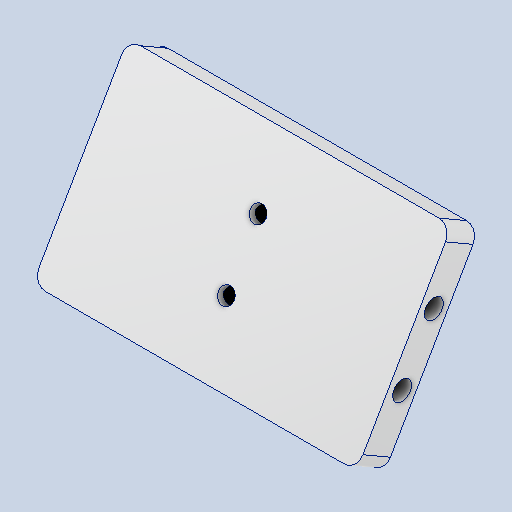
# Autodesk Inventor part: belt_liner_v5_Plate_4
Saved by Autodesk Inventor 2025.2 (Build 292293000, 293)
## iProperties
Created: 2025-02-23
Part Number: belt_liner_v5_Plate_4
Material: アルミニウム 6061
Document SubType Name: Modeling
Designer: haruy
Density: 2.7 g/cm^3
Appearance: アルミニウム - フラット
Author: haruy
Autodesk Inventor part; units mm, degrees
ref_plane "YZ Plane" through (0, 0, 0) normal (1, 0, 0) x (0, 1, 0)
ref_plane "XZ Plane" through (0, 0, 0) normal (0, 1, 0) x (-1, 0, 0)
ref_plane "XY Plane" through (0, 0, 0) normal (0, 0, 1) x (1, 0, 0)
derived "belt_liner_v5_Sketch_Base.ipt"
sketch "スケッチ1" plane through (300, 0, 0) normal (1, 0, 0) x (0, 1, 0)
  circle A0 centre (0, 0) radius 22.36
  circle A1 centre (742.4003, -428.625) radius 23.875 construction
  line L0 (0, 0) -> (0, -985.832)
  line L1 (0, 0) -> (742.4003, -428.625)
  line L2 (-48.7433, -24.4258) -> (-56.2433, -37.4162)
  line L3 (-56.2433, -37.4162) -> (725.7777, -488.9162)
  line L4 (725.7777, -488.9162) -> (733.2777, -475.9258)
  line L5 (733.2777, -475.9258) -> (-48.7433, -24.4258)
  line L6 (-44.1225, 123.2584) -> (-44.1225, 123.2584)
  line L7 (0, -985.832) -> (0, 0)
  circle A2 centre (0, 0) radius 12.5
  circle A3 centre (0, 0) radius 15
  line L8 (0, 0) -> (0, 0)
  circle A4 centre (0, 0) radius 24.06 construction
  line L9 (0, 0) -> (0, 0)
  line L10 (0, 0) -> (0, 0)
  line L11 (-48.7433, -24.4258) -> (-46.2433, -20.0957)
  circle A5 centre (742.4003, -428.625) radius 5
  line L12 (733.2777, -475.9258) -> (707.2969, -460.9258)
  line L13 (707.2969, -460.9258) -> (709.7969, -456.5957)
  line L14 (709.7969, -456.5957) -> (735.7777, -471.5957)
  line L15 (735.7777, -471.5957) -> (733.2777, -475.9258)
  circle A6 centre (738.0702, -426.125) radius 5.1
  line L16 (742.4003, -428.625) -> (509.0943, -293.9257)
  circle A7 centre (759.7208, -438.625) radius 5.1
  line L17 (740.6202, -421.7083) -> (762.2708, -434.2083)
  line L18 (735.5202, -430.5417) -> (757.1708, -443.0417)
  circle A8 centre (742.4003, -428.625) radius 22.175 construction
  circle A9 centre (738.0702, -426.125) radius 10.1 construction
  circle A10 centre (759.7208, -438.625) radius 10.1 construction
  line L19 (743.1202, -417.3781) -> (764.7708, -429.8781) construction
  line L20 (733.0202, -434.8719) -> (754.6708, -447.3719) construction
  line L21 (743.1202, -417.3781) -> (730.6598, -410.1842) construction
  line L22 (729.3233, -421.075) -> (734.3733, -412.3281) construction
  line L23 (764.7708, -429.8781) -> (770.9335, -433.4362) construction
  line L24 (770.9335, -433.4362) -> (771.2695, -433.6302)
  line L25 (754.6708, -447.3719) -> (764.7708, -429.8781)
  line L26 (764.7708, -429.8781) -> (773.431, -434.8781)
  line L27 (773.431, -434.8781) -> (763.331, -452.3719)
  line L28 (763.331, -452.3719) -> (754.6708, -447.3719) construction
  circle A11 centre (725.8674, -468.7607) radius 1.5
  circle A12 centre (0, 0) radius 30
  circle A13 centre (742.4003, -428.625) radius 6 construction
  circle A14 centre (0, 0) radius 24.06 construction
  circle A15 centre (0, 0) radius 24.06
  circle A16 centre (742.4003, -428.625) radius 24.06
  line L29 (754.4303, -407.7884) -> (12.03, 20.8366)
  circle A17 centre (725.8592, -419.075) radius 4
  circle A18 centre (725.8592, -419.075) radius 1.5
  circle A19 centre (742.4003, -428.625) radius 18.525 construction
  circle A20 centre (748.9869, -417.4167) radius 4
  line L30 (737.4369, -437.4219) -> (742.4869, -428.675)
  circle A21 centre (748.9869, -417.4167) radius 1.5
  line L31 (734.3733, -412.3281) -> (737.8233, -406.3526) construction
  line L32 (737.8233, -406.3526) -> (776.881, -428.9026)
  line L33 (773.431, -434.8781) -> (776.881, -428.9026)
  line L34 (737.8233, -406.3526) -> (723.6503, -415.7402)
  line L35 (720.8233, -435.7974) -> (759.881, -458.3474)
  line L36 (720.8233, -435.7974) -> (721.8667, -418.8295)
  line L37 (763.331, -452.3719) -> (759.881, -458.3474)
  circle A22 centre (735.9869, -439.9333) radius 4
  circle A23 centre (735.9869, -439.9333) radius 1.5
  circle A24 centre (717.2072, -463.7607) radius 1.5
  circle A25 centre (742.4003, -428.625) radius 34.06
  circle A26 centre (742.4869, -428.675) radius 8.5
  line L38 (-57.9836, -13.421) -> (-72.9836, -13.421)
  line L39 (-72.9836, -13.421) -> (-72.9836, -353.421)
  line L40 (-72.9836, -353.421) -> (-57.9836, -353.421)
  line L41 (-57.9836, -353.421) -> (-57.9836, -13.421)
  line L42 (457.0164, -338.421) -> (-72.9836, -338.421)
  line L43 (-72.9836, -338.421) -> (-72.9836, -353.421)
  line L44 (-72.9836, -353.421) -> (457.0164, -353.421)
  line L45 (457.0164, -353.421) -> (457.0164, -338.421)
  line L46 (427.0164, -338.421) -> (427.0164, -353.421)
  line L47 (457.0164, -353.421) -> (491.0931, -353.421)
  line L48 (491.0931, -353.421) -> (498.5931, -340.4306)
  line L49 (246.7786, -212.3659) -> (254.2786, -199.3755)
  line L50 (-207.9836, 176.579) -> (-227.9836, 176.579)
  line L51 (-227.9836, 176.579) -> (-227.9836, -413.421)
  line L52 (-227.9836, -413.421) -> (-207.9836, -413.421)
  line L53 (-207.9836, -413.421) -> (-207.9836, 176.579)
  line L54 (-52.0815, -339.4226) -> (-53.6411, -349.3003)
  line L55 (-53.6411, -349.3003) -> (703.9845, -468.9194)
  line L56 (703.9845, -468.9194) -> (705.5441, -459.0417)
  line L57 (705.5441, -459.0417) -> (-52.0815, -339.4226)
  circle A27 centre (0, 0) radius 24.06
  line L58 (1412.7204, 281.579) -> (-606.6364, 281.579)
  line L59 (1185.5776, -518.421) -> (-909.402, -518.421)
  line L60 (9.7721, 46.9258) -> (885.3238, -458.5742)
  line L61 (885.3238, -458.5742) -> (892.8238, -445.5838)
  line L62 (892.8238, -445.5838) -> (17.2721, 59.9162)
  line L63 (17.2721, 59.9162) -> (9.7721, 46.9258)
  line L64 (32.4276, 51.1662) -> (872.4722, -433.8338)
  line L65 (872.4722, -433.8338) -> (876.2222, -427.3386)
  line L66 (876.2222, -427.3386) -> (36.1776, 57.6614)
  line L67 (36.1776, 57.6614) -> (32.4276, 51.1662)
  line L68 (36.1776, 57.6614) -> (94.8941, 23.7614)
  line L69 (94.8941, 23.7614) -> (97.6441, 28.5245)
  line L70 (97.6441, 28.5245) -> (38.9276, 62.4245)
  line L71 (38.9276, 62.4245) -> (36.1776, 57.6614)
  circle A28 centre (215.5519, 104.2106) radius 120
  line L72 (-37.9836, 123.579) -> (-57.9836, 123.579)
  line L73 (-57.9836, 123.579) -> (-57.9836, 103.579)
  line L74 (-57.9836, 103.579) -> (-37.9836, 103.579)
  line L75 (-37.9836, 103.579) -> (-37.9836, 123.579)
  line L76 (215.5519, 104.2106) -> (184.4936, 220.1217)
  line L77 (215.5519, 104.2106) -> (99.6408, 73.1523)
  line L78 (215.5519, 104.2106) -> (155.5519, 0.2876)
  line L79 (187.4936, 225.3179) -> (96.6408, 67.9562)
  line L80 (96.6408, 67.9562) -> (91.4447, 70.9562)
  line L81 (91.4447, 70.9562) -> (182.2975, 228.3179)
  line L82 (182.2975, 228.3179) -> (187.4936, 225.3179)
  line L83 (182.2975, 228.3179) -> (179.2975, 223.1217)
  line L84 (179.2975, 223.1217) -> (174.9674, 225.6217)
  line L85 (174.9674, 225.6217) -> (177.9674, 230.8179)
  line L86 (177.9674, 230.8179) -> (182.2975, 228.3179)
  line L87 (91.4447, 70.9562) -> (94.4447, 76.1523)
  line L88 (94.4447, 76.1523) -> (90.1146, 78.6523)
  line L89 (90.1146, 78.6523) -> (87.1146, 73.4562)
  line L90 (87.1146, 73.4562) -> (91.4447, 70.9562)
  line L91 (-37.9836, 123.579) -> (2.0164, 123.579)
  line L92 (2.0164, 123.579) -> (2.0164, 103.579)
  line L93 (2.0164, 103.579) -> (-37.9836, 103.579)
  line L94 (-37.9836, 103.579) -> (-37.9836, 123.579)
  circle A29 centre (215.5519, 104.2106) radius 132.0681
  line L95 (101.1776, 170.2447) -> (38.9276, 62.4245)
  line L96 (32.4276, 51.1662) -> (11.6951, 15.2564)
  line L97 (11.6951, 15.2564) -> (20.3553, 10.2564)
  line L98 (20.3553, 10.2564) -> (41.0878, 46.1662)
  line L99 (41.0878, 46.1662) -> (32.4276, 51.1662)
  line L100 (149.5179, -10.1638) -> (155.5519, 0.2876)
  line L101 (149.5179, -10.1638) -> (20.3553, 10.2564)
  line L102 (79.4739, 0.91) -> (82.9739, 6.9722)
  line L103 (82.9739, 6.9722) -> (98.7532, -2.138)
  line L104 (179.2975, 223.1217) -> (151.7911, 205.8696)
  line L105 (94.4447, 76.1523) -> (95.6322, 108.5996)
  line L106 (96.6408, 67.9562) -> (113.8929, 40.4498)
  line L107 (-324.9836, 281.579) -> (-324.9836, -518.421)
  line L108 (1175.0164, 281.579) -> (1175.0164, -518.421)
  line L109 (17.2721, 59.9162) -> (9.7721, 46.9258)
  line L110 (9.7721, 46.9258) -> (-3.2183, 54.4258)
  line L111 (-3.2183, 54.4258) -> (4.2817, 67.4162)
  line L112 (4.2817, 67.4162) -> (17.2721, 59.9162)
  line L113 (-3.2183, 54.4258) -> (-5.7183, 50.0957)
  line L114 (-5.7183, 50.0957) -> (22.4276, 33.8457)
  line L115 (22.4276, 33.8457) -> (24.9276, 38.1758)
  line L116 (24.9276, 38.1758) -> (-3.2183, 54.4258)
  line L117 (-48.7433, -24.4258) -> (-46.2433, -20.0957)
  line L118 (-46.2433, -20.0957) -> (5.7183, -50.0957)
  line L119 (5.7183, -50.0957) -> (3.2183, -54.4258)
  line L120 (3.2183, -54.4258) -> (-48.7433, -24.4258)
  line L121 (789.6086, -403.313) -> (798.2689, -408.313)
  line L122 (798.2689, -408.313) -> (785.0364, -431.2324)
  line L123 (785.0364, -431.2324) -> (776.3761, -426.2324)
  line L124 (776.3761, -426.2324) -> (789.6086, -403.313)
  line L125 (885.3238, -458.5742) -> (882.8238, -462.9043)
  line L126 (882.8238, -462.9043) -> (856.843, -447.9043)
  line L127 (856.843, -447.9043) -> (859.343, -443.5742)
  line L128 (859.343, -443.5742) -> (885.3238, -458.5742)
  line L129 (7.6071, 48.1758) -> (11.9372, 45.6758)
  line L130 (11.9372, 45.6758) -> (19.4372, 58.6662)
  line L131 (19.4372, 58.6662) -> (15.1071, 61.1662)
  line L132 (15.1071, 61.1662) -> (7.6071, 48.1758)
  line L133 (19.4372, 58.6662) -> (14.4372, 50.0059)
  line L134 (14.4372, 50.0059) -> (24.8295, 44.0059)
  line L135 (24.8295, 44.0059) -> (29.8295, 52.6662)
  line L136 (29.8295, 52.6662) -> (19.4372, 58.6662)
  line L137 (931.2231, -485.0742) -> (935.5533, -487.5742)
  line L138 (935.5533, -487.5742) -> (951.5533, -459.8614)
  line L139 (951.5533, -459.8614) -> (947.2231, -457.3614)
  line L140 (947.2231, -457.3614) -> (931.2231, -485.0742)
  line L141 (944.4731, -462.1245) -> (934.9731, -478.579)
  line L142 (934.9731, -478.579) -> (919.3847, -469.579)
  line L143 (919.3847, -469.579) -> (928.8847, -453.1245)
  line L144 (928.8847, -453.1245) -> (944.4731, -462.1245)
  line L145 (924.1347, -461.3518) -> (939.7231, -470.3518)
  line L146 (926.6347, -457.0216) -> (921.6347, -465.6819)
  line L147 (921.6347, -465.6819) -> (882.6635, -443.1819)
  line L148 (882.6635, -443.1819) -> (887.6635, -434.5216)
  line L149 (887.6635, -434.5216) -> (926.6347, -457.0216)
  line L150 (888.9135, -432.3566) -> (881.4135, -445.347)
  line L151 (881.4135, -445.347) -> (874.4853, -441.347)
  line L152 (874.4853, -441.347) -> (881.9853, -428.3566)
  line L153 (881.9853, -428.3566) -> (888.9135, -432.3566)
  line L154 (31.0795, 54.8313) -> (23.5795, 41.8409)
  line L155 (23.5795, 41.8409) -> (30.5077, 37.8409)
  line L156 (30.5077, 37.8409) -> (38.0077, 50.8313)
  line L157 (38.0077, 50.8313) -> (31.0795, 54.8313)
  line L158 (16.9372, 54.3361) -> (27.3295, 48.3361)
  circle A30 centre (4.192, 47.2607) radius 1.25
  circle A31 centre (12.8522, 42.2607) radius 1.25
  line L159 (17.2721, 59.9162) -> (9.7721, 46.9258)
  line L160 (885.3238, -458.5742) -> (882.8238, -462.9043)
  line L161 (882.8238, -462.9043) -> (933.0533, -491.9043)
  line L162 (933.0533, -491.9043) -> (935.5533, -487.5742)
  line L163 (935.5533, -487.5742) -> (885.3238, -458.5742)
  line L164 (375.0164, 281.579) -> (375.0164, -518.421)
  line L165 (38.9276, 62.4245) -> (41.4276, 66.7546)
  line L166 (41.4276, 66.7546) -> (100.1441, 32.8546)
  line L167 (100.1441, 32.8546) -> (97.6441, 28.5245)
  line L168 (97.6441, 28.5245) -> (38.9276, 62.4245)
  line L169 (97.7242, 18.6633) -> (115.0447, 8.6633)
  line L170 (115.0447, 8.6633) -> (117.5447, 12.9934)
  line L171 (117.5447, 12.9934) -> (100.2242, 22.9934)
  line L172 (100.2242, 22.9934) -> (97.7242, 18.6633)
  line L173 (116.2947, 10.8284) -> (98.9742, 20.8284)
  line L174 (457.0164, -338.421) -> (465.1124, -338.421)
  line L175 (465.1124, -338.421) -> (472.6124, -325.4306)
  line L176 (-48.7433, -24.4258) -> (-56.2433, -37.4162)
  line L177 (-56.2433, -37.4162) -> (-77.8939, -24.9162)
  line L178 (-77.8939, -24.9162) -> (-70.3939, -11.9258)
  line L179 (-70.3939, -11.9258) -> (-48.7433, -24.4258)
  line L180 (-207.9836, -73.421) -> (-72.9836, -73.421)
  line L181 (-72.9836, -73.421) -> (-72.9836, -93.421)
  line L182 (-72.9836, -93.421) -> (-207.9836, -93.421)
  line L183 (-207.9836, -93.421) -> (-207.9836, -73.421)
  line L184 (-72.9836, -273.421) -> (-207.9836, -273.421)
  line L185 (-207.9836, -273.421) -> (-207.9836, -293.421)
  line L186 (-207.9836, -293.421) -> (-72.9836, -293.421)
  line L187 (-72.9836, -293.421) -> (-72.9836, -273.421)
  line L188 (-227.9836, -118.421) -> (-207.9836, -118.421)
  circle A32 centre (-30.1728, -32.2607) radius 1.25
  circle A33 centre (-12.8522, -42.2607) radius 1.25
  line L189 (-5.7183, 50.0957) -> (-46.2433, -20.0957)
  circle A34 centre (44.6769, 5.3827) radius 15
  circle A35 centre (17.6769, -41.3827) radius 15
  circle A36 centre (44.6769, 5.3827) radius 22
  circle A37 centre (17.6769, -41.3827) radius 22
  circle A38 centre (31.1769, -18) radius 3
  line L190 (44.6769, 5.3827) -> (17.6769, -41.3827)
  circle A39 centre (26.7448, 25.5678) radius 3
  circle A40 centre (-8.77, -35.9456) radius 3
  circle A41 centre (866.7533, -450.7393) radius 1.25
  circle A42 centre (875.4135, -455.7393) radius 1.25
  circle A43 centre (992.3767, -344.2894) radius 120
  line L191 (275.5519, 208.1337) -> (1052.3767, -240.3663)
  line L192 (-207.9836, -118.421) -> (1175.0164, -118.421)
  point P0 (730.6598, -410.1842)
  point P1 (-65.4836, -23.421)
  point P2 (-65.4836, -345.921)
  point P3 (447.0164, -345.921)
  point P4 (437.0164, -345.921)
  point P5 (477.5143, -336.921)
  point P6 (486.1745, -341.921)
  point P7 (-42.9836, -345.921)
  point P8 (694.8867, -462.421)
  point P9 (-57.9836, 113.579)
  point P10 (782.9924, -414.7727)
  point P11 (931.9289, -465.8518)
extrude "押し出し1" add sketch "スケッチ1" against normal blind 51 contours L13 L14 L15 L5
sketch "スケッチ2" plane through (249, 735.7777, -471.5957) normal (0, 0.5, 0.8660254) x (1, 0, 0)
  line L0 (0, -30) -> (0, 0) projected
  line L1 (51, -30) -> (0, -30) projected
  point P0 (-249, -873)
  point P1 (25.5, -20)
  point P2 (25.5, -10)
  dimension "d3" = 25.5
  dimension "d4" = 25.5
  dimension "d5" = 10
  dimension "d6" = 10
  measures "d3" distance from line of L0 point (25.5, -10)
  measures "d4" distance from line of point (25.5, -20) L0
  measures "d5" distance from line of point (25.5, -20) L1
  measures "d6" distance of point (25.5, -10) point (25.5, -20)
hole "穴1" at (274.5, 718.4572, -461.5957) at (274.5, 727.1174, -466.5957) direction (0, -0.5, -0.8660254) diameter 2.5 end through all
fillet "フィレット1" radius 2 4 edges at (300, 734.5277, -473.7607) (300, 708.5469, -458.7607) (249, 708.5469, -458.7607) (249, 734.5277, -473.7607)
equation "\"d4\" = d3"
equation "\"d6\" = d5"
